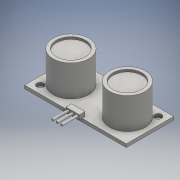
# Autodesk Inventor part: UltrasonicDistanceSencor
Saved by Autodesk Inventor 2016 (Build 200138000, 138)
## iProperties
Created: 2016-11-11
Part Number: UltrasonicDistanceSencor
Material: 一般
Document SubType Name: Modeling
Designer: Daisuke
Density: 1 g/cm^3
Appearance: 既定
Author: Daisuke
Autodesk Inventor part; units mm, degrees
ref_plane "YZ Plane" through (0, 0, 0) normal (1, 0, 0) x (0, 1, 0)
ref_plane "XZ Plane" through (0, 0, 0) normal (0, 1, 0) x (-1, 0, 0)
ref_plane "XY Plane" through (0, 0, 0) normal (0, 0, 1) x (1, 0, 0)
sketch "スケッチ1" plane through (0, 0, 0) normal (0, 0, 1) x (1, 0, 0)
  line L0 (0, 0) -> (45.7, 0)
  line L1 (45.7, 0) -> (45.7, 21.3)
  line L2 (45.7, 21.3) -> (0, 21.3)
  line L3 (0, 21.3) -> (0, 0)
  line L4 (45.7, 21.3) -> (42.2, 21.3) construction
  line L5 (42.2, 21.3) -> (42.2, 17.8) construction
  line L6 (42.2, 17.8) -> (45.7, 17.8) construction
  line L7 (45.7, 17.8) -> (45.7, 21.3) construction
  line L8 (0, 0) -> (3.5, 0) construction
  line L9 (3.5, 0) -> (3.5, 3.5) construction
  line L10 (3.5, 3.5) -> (0, 3.5) construction
  line L11 (0, 3.5) -> (0, 0) construction
  circle A0 centre (3.5, 3.5) radius 1.55
  circle A1 centre (42.2, 17.8) radius 1.55
  dimension "d0" = 45.7
  dimension "d1" = 21.3
  dimension "d2" = 3.5
  dimension "d3" = 3.5
  dimension "d4" = 3.5
  dimension "d5" = 3.5
  dimension "d6" = 3.1
  dimension "d7" = 3.1
  constraints: 24 end point, 6 parallel, 3 horizontal, 3 perpendicular, 2 centre point, 2 coincident
  measures "d0" distance of L2.end L1.end
  measures "d1" distance of L1.end L0.end
  measures "d2" distance of L6.end L5.end
  measures "d3" distance of L5.end L4.end
  measures "d4" distance of L10.end L9.end
  measures "d5" distance of L9.end L8.end
  measures "d6" diameter of A0
  measures "d7" diameter of A1
extrude "押し出し1" add sketch "スケッチ1" along normal blind 1.5
sketch "スケッチ2" plane through (0, 0, 1.5) normal (0, 0, 1) x (1, 0, 0)
  line L0 (0, 21.3) -> (0, 0) construction
  line L1 (0, 10.65) -> (2, 10.65) construction
  line L2 (2, 10.65) -> (18.3, 10.65) construction
  line L3 (18.3, 10.65) -> (27.4, 10.65) construction
  line L4 (27.4, 10.65) -> (43.7, 10.65) construction
  line L5 (43.7, 10.65) -> (45.7, 10.65) construction
  circle A0 centre (10.15, 10.65) radius 8
  circle A1 centre (35.55, 10.65) radius 8
  dimension "d10" = 2
  dimension "d11" = 16.3
  dimension "d12" = 9.1
  dimension "d13" = 16.3
  dimension "d14" = 2
  dimension "d15" = 16
  dimension "d16" = 16
  constraints: 10 end point, 4 point on line, 3 midpoint, 2 centre point, 1 horizontal
  measures "d10" distance of L1.start L1.end
  measures "d11" distance of L1.end L2.end
  measures "d12" distance of L2.end L3.end
  measures "d13" distance of L3.end L4.end
  measures "d14" distance of L4.end L5.end
  measures "d15" diameter of A0
  measures "d16" diameter of A1
extrude "押し出し2" add sketch "スケッチ2" along normal blind 14
sketch "スケッチ3" plane through (10.15, 10.65, 15.5) normal (0, 0, 1) x (1, 0, 0)
  circle A0 centre (0, 0) radius 6.5
  circle A1 centre (25.4, 0) radius 8 projected
  circle A2 centre (25.4, 0) radius 6.5
  point P0 (-10.15, -10.65)
  dimension "d19" = 13
  dimension "d20" = 13
  constraints: 2 centre point, 1 coincident
  measures "d19" diameter of A0
  measures "d20" diameter of A2
extrude "押し出し3" cut sketch "スケッチ3" against normal blind 1 contours A0 | A2
sketch "スケッチ4" plane through (0, 0, 1.5) normal (0, 0, 1) x (1, 0, 0)
  line L0 (19.85, -1.25) -> (25.85, -1.25)
  line L1 (25.85, -1.25) -> (25.85, 1.25)
  line L2 (25.85, 1.25) -> (19.85, 1.25)
  line L3 (19.85, 1.25) -> (19.85, -1.25)
  line L4 (0, 0) -> (45.7, 0) projected
  line L5 (19.85, -1.25) -> (25.85, 1.25) construction
  line L6 (25.85, -1.25) -> (19.85, 1.25) construction
  point P0 (22.85, 0)
  dimension "d23" = 6
  dimension "d24" = 2.5
  constraints: 12 end point, 3 midpoint, 2 parallel, 1 horizontal, 1 perpendicular
  measures "d23" distance of L2.end L1.end
  measures "d24" distance of L1.end L0.end
extrude "押し出し4" add sketch "スケッチ4" along normal blind 2
sketch "スケッチ5" plane through (19.85, -1.25, 1.5) normal (0, -1, 0) x (1, 0, 0)
  circle A0 centre (3, 1) radius 0.5
  line L0 (0, 0) -> (0, 2) construction
  line L1 (0, 1) -> (1, 1) construction
  line L2 (6, 0) -> (6, 2) construction
  line L3 (6, 1) -> (5, 1) construction
  circle A1 centre (1, 1) radius 0.5
  circle A2 centre (5, 1) radius 0.5
  point P0 (-19.85, -1.5)
  dimension "d27" = 1
  dimension "d28" = 1
  dimension "d29" = 1
  dimension "d30" = 1
  dimension "d31" = 1
  constraints: 4 end point, 3 centre point, 2 coincident, 2 horizontal, 2 midpoint
  measures "d27" diameter of A0
  measures "d28" distance of L1.start L1.end
  measures "d29" distance of L3.start L3.end
  measures "d30" diameter of A1
  measures "d31" diameter of A2
extrude "押し出し5" add sketch "スケッチ5" along normal blind 7
